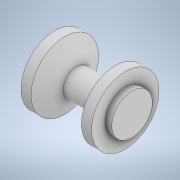
# Autodesk Inventor part: Ch3 Part 3
Saved by Autodesk Inventor 2020 (Build 240168000, 168)
## iProperties
Created: 2021-02-04
Part Number: Ch3 Part 3
Material: Generic
Document SubType Name: Modeling
Designer: austi
Density: 1 g/cm^3
Appearance: Default
Author: austi
Autodesk Inventor part; units mm, degrees
ref_plane "YZ Plane" through (0, 0, 0) normal (1, 0, 0) x (0, 1, 0)
ref_plane "XZ Plane" through (0, 0, 0) normal (0, 1, 0) x (-1, 0, 0)
ref_plane "XY Plane" through (0, 0, 0) normal (0, 0, 1) x (1, 0, 0)
sketch "Sketch1" plane through (0, 0, 0) normal (0, 0, 1) x (1, 0, 0)
  line L0 (0, 25.4) -> (-25.4, 25.4)
  line L1 (-25.4, 25.4) -> (-47.397, 63.5)
  line L2 (-47.397, 63.5) -> (-66.447, 63.5)
  line L3 (-66.447, 63.5) -> (-66.447, 38.1)
  line L4 (-66.447, 38.1) -> (-79.147, 38.1)
  line L5 (0, -12.7) -> (0, 76.2) projected
  line L6 (-110.8059, 0) -> (110.8059, 0) projected
  line L7 (0, 25.4) -> (25.4, 25.4)
  line L8 (25.4, 25.4) -> (47.397, 63.5)
  line L9 (47.397, 63.5) -> (66.447, 63.5)
  line L10 (66.447, 63.5) -> (66.447, 38.1)
  line L11 (66.447, 38.1) -> (79.147, 38.1)
  line L12 (79.147, 38.1) -> (79.147, 0)
  line L13 (-79.147, 38.1) -> (-79.147, 0)
  line L14 (-79.147, 0) -> (79.147, 0)
  point P0 (0, 0)
  dimension "d3" = 19.05
  dimension "d13" = 60
  dimension "d14" = 12.7
  dimension "d15" = 127
  dimension "d16" = 76.2
  dimension "d17" = 50.8
  dimension "d18" = 50.8
  constraints: 26 end point, 4 perpendicular, 3 equal length, 2 collinear, 2 horizontal, 2 parallel, 1 horizontal alignment, 1 vertical, 5 other
  measures "d3" distance of L1.end L2.end
  measures "d13" angle of L8 L1
  measures "d14" distance of L3.end L4.end
  measures "d15" diameter of L9.end L14
  measures "d16" diameter of L11.end L14
  measures "d17" diameter of L7.end L14
  measures "d18" distance of L7.end L0.end
revolve "Revolution1" add sketch "Sketch1" angle 360 about axis through (-79.147, 0, 0) along (1, 0, 0)
body "Solid1"
